# Autodesk Inventor part: Bottom Mold_Remote Bottom_WP
Saved by Autodesk Inventor 2016 (Build 200138000, 138)
## iProperties
Created: 2015-07-09
Part Number: Bottom Mold_Remote Bottom_WP
Material: Generic
Document SubType Name: Modeling
Designer: Samuel Clay
Density: 1 g/cm^3
Appearance: Default
Author: Samuel Clay
d0: -0.750 in
d1: 1.250 in
d2: 1.250 in
d3: 1.250 in
d4: 1.250 in
d5: 1.500 in
d6: 0.00 deg
Xmin: -1.250 in
Ymin: -1.250 in
Zmin: -0.750 in
Xmax: 1.250 in
Ymax: 1.250 in
Zmax: 0.750 in
Autodesk Inventor part; units mm, degrees
ref_plane "YZ Plane" through (0, 0, 0) normal (1, 0, 0) x (0, 1, 0)
ref_plane "XZ Plane" through (0, 0, 0) normal (0, 1, 0) x (-1, 0, 0)
ref_plane "XY Plane" through (0, 0, 0) normal (0, 0, 1) x (1, 0, 0)
sketch "Sketch1" plane through (0, 0, -19.05) normal (0, 0, 1) x (1, 0, 0)
  line L0 (-31.75, 31.75) -> (31.75, 31.75)
  line L1 (31.75, 31.75) -> (31.75, -31.75)
  line L2 (31.75, -31.75) -> (-31.75, -31.75)
  line L3 (-31.75, -31.75) -> (-31.75, 31.75)
  point P0 (0, 0)
  dimension "d1" = 31.75
  dimension "d2" = 31.75
  dimension "d3" = 31.75
  dimension "d4" = 31.75
  constraints: 8 end point, 2 parallel, 1 horizontal, 1 perpendicular, 1 other
  measures "d1" distance from line of L3 point (0, 0)
  measures "d2" distance from line of L1 point (0, 0)
  measures "d3" distance from line of L2 point (0, 0)
  measures "d4" distance from line of L0 point (0, 0)
extrude "Extrusion1" add sketch "Sketch1" along normal blind 38.1
equation "\"d1\" = -Xmin"
equation "\"d2\" = Xmax"
equation "\"d3\" = -Ymin"
equation "\"d4\" = Ymax"
equation "\"d5\" = Zmax - Zmin"
equation "\"Xmin\" = -31.75"
equation "\"Ymin\" = -31.75"
equation "\"Zmin\" = -19.05"
equation "\"Xmax\" = 31.75"
equation "\"Ymax\" = 31.75"
equation "\"Zmax\" = 19.05"
body "Solid1"
